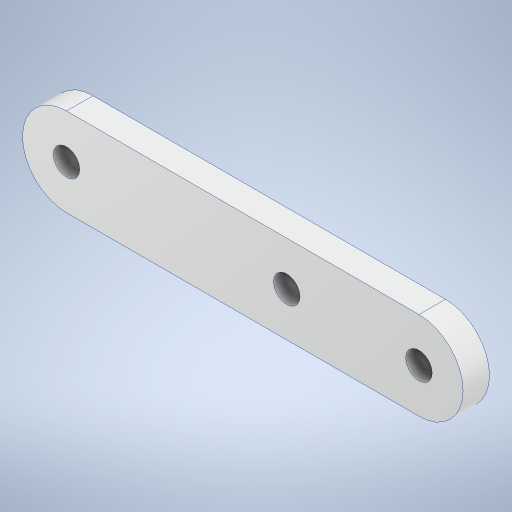
# Autodesk Inventor part: Arm3
Saved by Autodesk Inventor 2023 (Build 270158000, 158)
## iProperties
Created: 2024-02-06
Part Number: Arm3
Material: Aluminum 6061
Document SubType Name: Modeling
Designer: victo
Density: 2.7 g/cm^3
Appearance: Aluminum - Flat
Author: victo
Autodesk Inventor part; units mm, degrees
ref_plane "YZ Plane" through (0, 0, 0) normal (1, 0, 0) x (0, 1, 0)
ref_plane "XZ Plane" through (0, 0, 0) normal (0, 1, 0) x (-1, 0, 0)
ref_plane "XY Plane" through (0, 0, 0) normal (0, 0, 1) x (1, 0, 0)
sketch "Sketch1" plane through (0, 0, 0) normal (0, 0, 1) x (1, 0, 0)
  line L0 (0, 0) -> (40, 0) construction
  line L1 (0, -5) -> (40, -5)
  line L2 (40, 5) -> (0, 5)
  arc A0 (0, 5) -> (0, -5) centre (0, 0) ccw
  arc A1 (40, -5) -> (40, 5) centre (40, 0) ccw
  line L3 (0, 0) -> (40, 0) construction
  circle A2 centre (0, 0) radius 1.5
  circle A3 centre (40, 0) radius 1.5
  circle A4 centre (25, 0) radius 1.5
  point P0 (20, 0)
  dimension "d0" = 40
  dimension "d1" = 0
  dimension "d2" = 10
  dimension "d3" = 3
  dimension "d4" = 3
  dimension "d5" = 3
  dimension "d6" = 15
  constraints: 10 end point, 5 centre point, 4 point on circle, 4 tangent, 2 coincident, 2 horizontal, 1 collinear, 1 midpoint, 1 parallel, 1 point on line
  measures "d0" distance of L0.start L0.end
  measures "d1" distance between parallel lines of L0 L3
  measures "d2" diameter of A1
  measures "d3" diameter of A2
  measures "d4" diameter of A3
  measures "d5" diameter of A4
  measures "d6" distance of A4.centre L0.end
extrude "Extrusion1" add sketch "Sketch1" along normal blind 3
body "Solid1"
